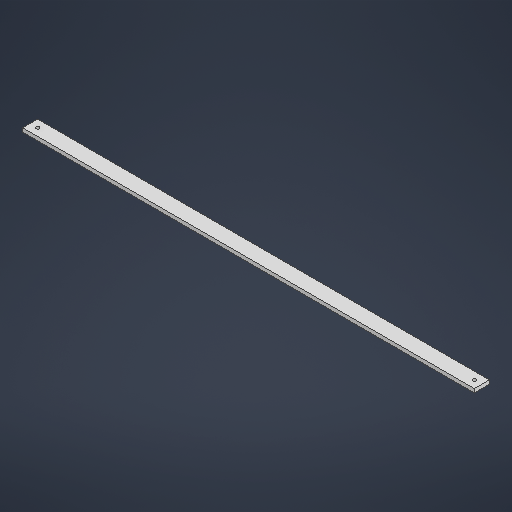
# Autodesk Inventor part: gpu_support
Saved by Autodesk Inventor 2026.2 (Build 302298010, 298A)
## iProperties
Created: 2026-05-31
Part Number: gpu_support
Material: 一般
Document SubType Name: Modeling
Designer: nyxeon
Density: 1 g/cm^3
Appearance: 既定
Author: nyxeon
Autodesk Inventor part; units mm, degrees
ref_plane "YZ Plane" through (0, 0, 0) normal (1, 0, 0) x (0, 1, 0)
ref_plane "XZ Plane" through (0, 0, 0) normal (0, 1, 0) x (-1, 0, 0)
ref_plane "XY Plane" through (0, 0, 0) normal (0, 0, 1) x (1, 0, 0)
sketch "スケッチ1" plane through (0, 0, 0) normal (0, 1, 0) x (-1, 0, 0)
  line L0 (300, 10) -> (-300, 10)
  line L1 (-300, 10) -> (-300, -10)
  line L2 (-300, -10) -> (300, -10)
  line L3 (300, -10) -> (300, 10)
  circle A0 centre (290, 0) radius 2.25
  circle A1 centre (-290, 0) radius 2.25
  point P0 (0, 0)
  point P1 (0, 10)
  point P2 (300, 0)
  point P3 (-300, 0)
  dimension "d0" = 20
  dimension "d1" = 600
  dimension "d2" = 4.5
  dimension "d3" = 10
  dimension "d4" = 10
  constraints: 8 end point, 3 horizontal alignment, 3 midpoint, 2 centre point, 2 parallel, 1 equal radius, 1 horizontal, 1 perpendicular, 1 vertical alignment
  measures "d0" distance of L2.end L0.start
  measures "d1" distance of L0.start L0.end
  measures "d2" diameter of A0
  measures "d3" distance from line of A0.centre L3
  measures "d4" distance of point (-300, 0) A1.centre
extrude "押し出し1" add sketch "スケッチ1" along normal blind 5
equation "\"d4\" = d3"
